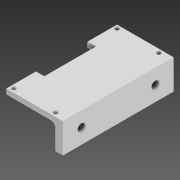
# Autodesk Inventor part: Ultrasonic_holder
Saved by Autodesk Inventor 2020 (Build 240168000, 168)
## iProperties
Created: 2022-08-18
Part Number: Ultrasonic_holder
Material: Generic
Document SubType Name: Modeling
Designer: Umair
Density: 1 g/cm^3
Appearance: Default
Author: Umair
Autodesk Inventor part; units mm, degrees
ref_plane "YZ Plane" through (0, 0, 0) normal (1, 0, 0) x (0, 1, 0)
ref_plane "XZ Plane" through (0, 0, 0) normal (0, 1, 0) x (-1, 0, 0)
ref_plane "XY Plane" through (0, 0, 0) normal (0, 0, 1) x (1, 0, 0)
sketch "Sketch1" plane through (0, 0, 0) normal (0, 1, 0) x (-1, 0, 0)
  line L0 (10, 22.5) -> (-10, 22.5)
  line L1 (-10, 22.5) -> (-10, -22.5)
  line L2 (-10, -22.5) -> (10, -22.5)
  line L3 (10, -22.5) -> (10, 22.5)
  line L4 (10, 22.5) -> (-10, -22.5) construction
  line L5 (-10, 22.5) -> (10, -22.5) construction
  line L6 (13.4184, 10.4917) -> (6.5816, 10.4917)
  line L7 (6.5816, 10.4917) -> (6.5816, -10.4917)
  line L8 (6.5816, -10.4917) -> (13.4184, -10.4917)
  line L9 (13.4184, -10.4917) -> (13.4184, 10.4917)
  line L10 (13.4184, 10.4917) -> (6.5816, -10.4917) construction
  line L11 (6.5816, 10.4917) -> (13.4184, -10.4917) construction
  line L12 (8.5, 21) -> (-8.5, 21)
  line L13 (-8.5, 21) -> (-8.5, -21)
  line L14 (-8.5, -21) -> (8.5, -21)
  line L15 (8.5, -21) -> (8.5, 21)
  line L16 (8.5, 21) -> (-8.5, -21) construction
  line L17 (-8.5, 21) -> (8.5, -21) construction
  circle A0 centre (8.5, 21) radius 0.75
  circle A1 centre (8.5, -21) radius 0.75
  circle A2 centre (-8.5, -21) radius 0.75
  circle A3 centre (-8.5, 21) radius 0.75
  point P0 (0, 0)
  point P1 (10, 0)
  point P2 (10, 10.4917)
  point P3 (10, -10.4917)
  dimension "d0" = 20
  dimension "d1" = 45
  dimension "d2" = 17
  dimension "d3" = 42
  dimension "d4" = 1.5
  dimension "d5" = 1.5
  dimension "d6" = 1.5
  dimension "d7" = 1.5
  constraints: 36 end point, 7 midpoint, 6 parallel, 4 centre point, 4 coincident, 3 horizontal, 3 perpendicular
  measures "d0" distance of L2.end L1.end
  measures "d1" distance of L1.end L0.end
  measures "d2" distance of L14.end L13.end
  measures "d3" distance of L13.end L12.end
  measures "d4" diameter of A0
  measures "d5" diameter of A1
  measures "d6" diameter of A2
  measures "d7" diameter of A3
extrude "Extrusion1" add sketch "Sketch1" along normal blind 2 contours L3 L6 L15 A0 L12 A3 L13 A2 L14 A1 L8 L2 L1 L0 | L6 L7 L8 L15 A1 L14 A2 L13 A3 L12 A0
sketch "Sketch2" plane through (0, 0, 0) normal (0, -1, 0) x (1, 0, 0)
  line L0 (10, -22.5) -> (-10, -22.5) projected
  line L1 (10, -22.5) -> (13, -22.5)
  line L2 (13, -22.5) -> (13, 22.5)
  line L3 (-10, 22.5) -> (10, 22.5) projected
  line L4 (13, 22.5) -> (10, 22.5)
  line L5 (10, 22.5) -> (10, -22.5)
  point P0 (0, 0)
  dimension "d10" = 3
  dimension "d11" = 45
  constraints: 8 end point, 1 horizontal, 1 perpendicular
  measures "d10" distance of L0.start L1.end
  measures "d11" distance of L1.end L2.end
extrude "Extrusion2" add sketch "Sketch2" along normal blind 10 and the other way blind 2
fillet "Fillet1" radius 2 1 edges at (10, 0, 0)
sketch "Sketch3" plane through (13, -10, 22.5) normal (1, 0, 0) x (0, 0, -1)
  line L0 (0, 0) -> (45, 0) projected
  line L1 (22.5, 0) -> (22.5, 5)
  line L2 (22.5, 5) -> (22.5, 6)
  line L3 (22.5, 6) -> (7.5, 6)
  line L4 (7.5, 6) -> (37.5, 6)
  circle A0 centre (37.5, 6) radius 1.5
  circle A1 centre (7.5, 6) radius 1.5
  point P0 (22.5, 10)
  dimension "d17" = 5
  dimension "d18" = 1
  dimension "d19" = 15
  dimension "d20" = 30
  dimension "d21" = 3
  dimension "d22" = 3
  constraints: 8 end point, 2 centre point, 2 coincident, 2 point on line, 1 midpoint, 1 perpendicular, 1 vertical
  measures "d17" distance of L1.start L1.end
  measures "d18" distance of L1.end L2.end
  measures "d19" distance of L2.end L3.end
  measures "d20" distance of L3.end L4.end
  measures "d21" diameter of A0
  measures "d22" diameter of A1
extrude "Extrusion3" cut sketch "Sketch3" against normal blind 10
body "Solid1"
